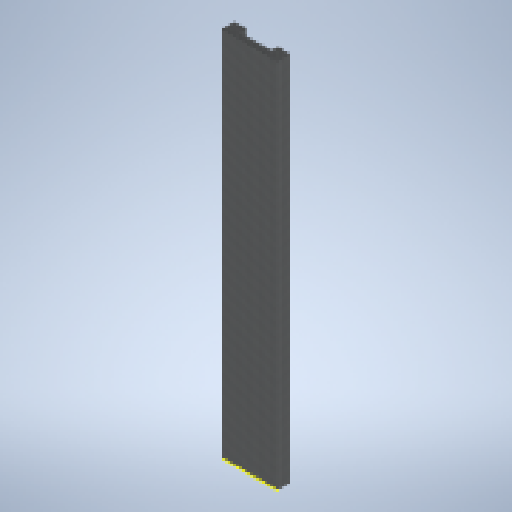
# Autodesk Inventor part: Part1
Saved by Autodesk Inventor 2023 (Build 270158000, 158)
## iProperties
Created: 2023-03-22
Part Number: Part1
Material: Generic
Document SubType Name: Modeling
Designer: sebas
Density: 1 g/cm^3
Appearance: Expanded Metal 01
Author: sebas
Autodesk Inventor part; units mm, degrees
ref_plane "YZ Plane" through (0, 0, 0) normal (1, 0, 0) x (0, 1, 0)
ref_plane "XZ Plane" through (0, 0, 0) normal (0, 1, 0) x (-1, 0, 0)
ref_plane "XY Plane" through (0, 0, 0) normal (0, 0, 1) x (1, 0, 0)
sketch "Sketch3" plane through (0, 0, 0) normal (0, 1, 0) x (-1, 0, 0)
  line L0 (0, 0) -> (-45, 0)
  line L1 (-45, 0) -> (-45, -10)
  line L2 (-35, -5) -> (-35, -10)
  line L3 (-35, -10) -> (-45, -10)
  line L4 (-35, -5) -> (-10, -5)
  line L5 (-10, -5) -> (-10, -10)
  line L6 (-10, -10) -> (0, -10)
  line L7 (0, -10) -> (0, 0)
  dimension "d1" = 45
  dimension "d2" = 10
  dimension "d7" = 25
  constraints: 16 end point, 3 horizontal, 2 perpendicular, 2 vertical
  measures "d1" distance of L0.start L0.end
  measures "d2" distance of L0.end L1.end
  measures "d7" distance of L4.end L2.start
extrude "Extrusion1" add sketch "Sketch3" along normal blind 300
sketch "Sketch5" plane through (0, 0, 0) normal (0, -1, 0) x (1, 0, 0)
  line L0 (0, 0) -> (45, 0) projected
body "Solid1"
